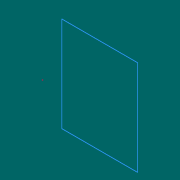
# Autodesk Inventor part: Stuze_Poti
Saved by Autodesk Inventor 2020.1 (Build 241239000, 239)
## iProperties
Created: 2020-01-27
Part Number: Stuze_Poti
Material: Generic
Document SubType Name: Modeling
Designer: Pluscrafter
Density: 1 g/cm^3
Appearance: Default
Author: Pluscrafter
Autodesk Inventor part; units mm, degrees
ref_plane "YZ Plane" through (0, 0, 0) normal (1, 0, 0) x (0, 1, 0)
ref_plane "XZ Plane" through (0, 0, 0) normal (0, 1, 0) x (-1, 0, 0)
ref_plane "XY Plane" through (0, 0, 0) normal (0, 0, 1) x (1, 0, 0)
sketch "Sketch1" plane through (0, 0, 0) normal (0, 0, 1) x (1, 0, 0)
  line L0 (42.4705, 38.9699) -> (30.2705, 38.9699)
  line L1 (20.2705, 28.9699) -> (20.2705, -23.0101)
  line L2 (52.4705, -23.0101) -> (52.4705, 28.9699)
  line L3 (31.4205, 33.9699) -> (41.3205, 33.9699)
  line L4 (41.3205, 33.9699) -> (41.3205, 22.1899)
  line L5 (41.3205, 22.1899) -> (31.4205, 22.1899)
  line L6 (31.4205, 22.1899) -> (31.4205, 33.9699)
  arc A0 (30.2705, 38.9699) -> (20.2705, 28.9699) centre (30.2705, 28.9699) ccw
  arc A1 (52.4705, 28.9699) -> (42.4705, 38.9699) centre (42.4705, 28.9699) ccw
  line L7 (31.3705, -23.0101) -> (31.3705, -20.0101)
  line L8 (31.3705, -20.0101) -> (41.3705, -20.0101)
  line L9 (41.3705, -20.0101) -> (41.3705, -23.0101)
  line L10 (20.2705, -23.0101) -> (31.3705, -23.0101)
  line L11 (41.3705, -23.0101) -> (52.4705, -23.0101)
  line L12 (41.3705, -23.0101) -> (41.3205, -23.0101)
  line L13 (31.4205, -23.0101) -> (31.3705, -23.0101)
  point P0 (0, 0)
  dimension "d0" = 9.9
  dimension "d1" = 11.78
  dimension "d3" = 32.2
  dimension "d5" = 11.15
  dimension "d6" = 5
  dimension "d7" = 10
  dimension "d8" = 10
  dimension "d9" = 3
  dimension "d10" = 11.1
  constraints: 28 end point, 8 parallel, 4 horizontal, 4 perpendicular, 4 point on circle, 4 tangent, 2 centre point, 2 point on line, 1 equal radius
  measures "d0" distance of L4.end L5.end
  measures "d1" distance of L3.end L4.end
  measures "d3" distance between parallel lines of L2 L1
  measures "d5" distance between parallel lines of L1 L6
  measures "d6" distance between parallel lines of L0 L3
  measures "d7" radius of A0
  measures "d8" distance of L7.end L8.end
  measures "d9" distance of L7.start L7.end
  measures "d10" distance between parallel lines of L1 L7
extrude "Extrusion1" add sketch "Sketch1" along normal blind 3
body "Solid1"
